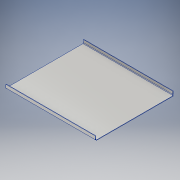
# Autodesk Inventor part: BellyPan
Saved by Autodesk Inventor 2016 (Build 200138000, 138)
## iProperties
Created: 2017-01-21
Part Number: BellyPan
Material: Aluminum 6061
Document SubType Name: Modeling
Designer: hamblettk
Density: 2.7 g/cm^3
Appearance: Aluminum - Flat
Author: hamblettk
Autodesk Inventor part; units mm, degrees
ref_plane "YZ Plane" through (0, 0, 0) normal (1, 0, 0) x (0, 1, 0)
ref_plane "XZ Plane" through (0, 0, 0) normal (0, 1, 0) x (-1, 0, 0)
ref_plane "XY Plane" through (0, 0, 0) normal (0, 0, 1) x (1, 0, 0)
sketch "Sketch2" plane through (0, 0, 0) normal (1, 0, 0) x (0, 1, 0)
  line L0 (0, 0) -> (0, -269.875)
  line L1 (0, 0) -> (0, 269.875)
  line L2 (0, 269.875) -> (25.4, 269.875)
  line L3 (0, -269.875) -> (25.4, -269.875)
  line L4 (25.4, -269.875) -> (25.4, -266.7)
  line L5 (25.4, 269.875) -> (25.4, 266.7)
  line L6 (25.4, 266.7) -> (3.175, 266.7)
  line L7 (25.4, -266.7) -> (3.175, -266.7)
  line L8 (3.175, -266.7) -> (3.175, 266.7)
  dimension "d10" = 269.875
  dimension "d11" = 269.875
  dimension "d12" = 25.4
  dimension "d13" = 25.4
  dimension "d14" = 3.175
  dimension "d15" = 3.175
  dimension "d16" = 22.225
  dimension "d17" = 22.225
  constraints: 18 end point, 4 vertical, 3 horizontal, 1 perpendicular
  measures "d10" distance of L0.start L0.end
  measures "d11" distance of L0.start L1.end
  measures "d12" distance of L1.end L2.end
  measures "d13" distance of L0.end L3.end
  measures "d14" distance of L3.end L4.end
  measures "d15" distance of L2.end L5.end
  measures "d16" distance of L5.end L6.end
  measures "d17" distance of L4.end L7.end
extrude "Extrusion2" add sketch "Sketch2" along normal blind 616.1532
fillet "Fillet1" radius 3.175 4 edges at (308.0766, 0, 269.875) (308.0766, 0, -269.875) (308.0766, 3.175, -266.7) (308.0766, 3.175, 266.7)
sketch "Sketch5" plane through (616.1532, 0, 0) normal (1, 0, 0) x (0, 0, -1)
  arc A0 (-269.875, 3.175) -> (-266.7, 0) centre (-266.7, 3.175) ccw projected
  line L0 (-266.7, 0) -> (-266.7, 3.175)
  line L1 (263.525, 3.175) -> (-263.525, 3.175) projected
  line L2 (-266.7, 3.175) -> (263.525, 3.175)
  line L3 (263.525, 3.175) -> (263.525, 0)
  line L4 (-266.7, 0) -> (266.7, 0) projected
  line L5 (263.525, 0) -> (-266.7, 0)
  point P0 (0, 0)
  constraints: 8 end point, 1 collinear, 1 horizontal, 1 perpendicular, 1 point on line, 1 tangent, 1 vertical
extrude "Extrusion6" add sketch "Sketch5" along normal blind 7.112
body "Solid2"
